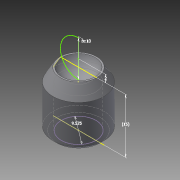
# Autodesk Inventor part: Rod End 9.5mm
Saved by Autodesk Inventor 2015 SP1 (Build 190203100, 203)
## iProperties
Created: 2015-04-29
Part Number: Rod End 9.5mm
Material: Generic
Document SubType Name: Modeling
Designer: tsmember
Density: 1 g/cm^3
Appearance: Default
Author: tsmember
Autodesk Inventor part; units mm, degrees
ref_plane "YZ Plane" through (0, 0, 0) normal (1, 0, 0) x (0, 1, 0)
ref_plane "XZ Plane" through (0, 0, 0) normal (0, 1, 0) x (-1, 0, 0)
ref_plane "XY Plane" through (0, 0, 0) normal (0, 0, 1) x (1, 0, 0)
sketch "RingSketch" plane through (0, 0, 0) normal (0, 0, 1) x (1, 0, 0)
  circle A0 centre (0, 0) radius 7
  dimension "RingDia" = 14
  constraints: 1 centre point, 1 coincident
  measures "RingDia" diameter of A0
extrude "Ring" add sketch "RingSketch" against normal blind 1
sketch "ShankSketch" plane through (0, 0, -1) normal (0, 0, -1) x (-1, 0, 0)
  circle A0 centre (0, 0) radius 7
  dimension "ShankDia" = 14
  constraints: 1 centre point, 1 coincident
  measures "ShankDia" diameter of A0
extrude "Shank" add sketch "ShankSketch" along normal blind 10.536
sketch "ConeSketch" plane through (0, 0, 0) normal (1, 0, 0) x (0, 1, 0)
  line L0 (0, 0) -> (7, 0)
  line L1 (7, 0) -> (5, 3.4641)
  line L2 (5, 3.4641) -> (0, 3.4641)
  line L3 (0, 3.4641) -> (0, 0)
  line L4 (-7, 0) -> (7, 0) projected
  dimension "ConeAngle" = 60
  dimension "ConeBase" = 7
  dimension "ConeTipDia" = 5
  constraints: 8 end point, 1 horizontal, 1 parallel, 1 perpendicular
  measures "ConeAngle" angle of L0 L1
  measures "ConeBase" distance of L0.start L0.end
  measures "ConeTipDia" distance of L1.end L2.end
revolve "Cone" add sketch "ConeSketch" angle 360 about axis through (0, 0, 3.4641) along (0, 0, -1)
sketch "SocketSketch" plane through (0, 0, 0) normal (0, 1, 0) x (-1, 0, 0)
  arc A0 (0, 0.4641) -> (0, 10.4641) centre (0, 5.4641) ccw
  line L0 (0, 10.4641) -> (0, 0.4641)
  line L1 (-5, 3.4641) -> (5, 3.4641) projected
  line L2 (5, 3.4641) -> (7, 0) projected
  point P0 (0, 0)
  dimension "RecessDia" = 10
  dimension "BallOffset" = 2
  constraints: 2 end point, 2 point on circle, 1 centre point, 1 vertical
  measures "RecessDia" diameter of A0
  measures "BallOffset" distance from line of L1 A0.centre
revolve "Socket" cut sketch "SocketSketch" angle 360 about axis through (0, 0, 10.4641) along (0, 0, -1)
sketch "MagnetHoleSketch" plane through (0, 0, -11.536) normal (0, 0, -1) x (-1, 0, 0)
  circle A0 centre (0, 0) radius 4.7625
  dimension "MagnetHoleDia" = 9.525
  constraints: 1 centre point, 1 coincident
  measures "MagnetHoleDia" diameter of A0
extrude "MagnetHole" cut sketch "MagnetHoleSketch" against normal blind 11.5001
sketch "PartLength" plane through (0, 0, 0) normal (0, 1, 0) x (-1, 0, 0)
  line L0 (-5, 3.4641) -> (5, 3.4641) projected
  line L1 (-7, -11.536) -> (7, -11.536) projected
  point P0 (0, 0)
  dimension "PartLen" = 15.0001
  measures "PartLen" distance between parallel lines of L1 L0
chamfer "Chamfer1" distance 1 angle 45 1 edges at (7, 0, -11.536)
equation "\"ShankDia\" = RingDia"
equation "\"ConeBase\" = 0.5 * RingDia"
equation "\"ConeTipDia\" = 0.5 * BallDia"
equation "\"RecessDia\" = BallDia"
equation "\"BallDia\" = 10"
body "Solid1"
